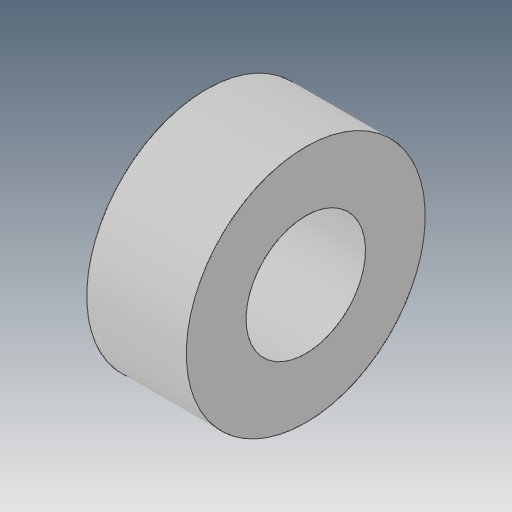
# Autodesk Inventor part: セットカラー_6mm
Saved by Autodesk Inventor 2019 (Build 230136000, 136)
## iProperties
Created: 2020-10-25
Part Number: セットカラー_6mm
Material: 一般
Document SubType Name: Modeling
Designer: zhept
Density: 1 g/cm^3
Appearance: 既定
Mass: 0.424115 g
Surface Area: 4.52389 cm^2
Volume: 0.424115 cm^3
Author: zhept
Autodesk Inventor part; units mm, degrees
ref_plane "YZ Plane" through (0, 0, 0) normal (1, 0, 0) x (0, 1, 0)
ref_plane "XZ Plane" through (0, 0, 0) normal (0, 1, 0) x (-1, 0, 0)
ref_plane "XY Plane" through (0, 0, 0) normal (0, 0, 1) x (1, 0, 0)
sketch "スケッチ1" plane through (0, 0, 0) normal (1, 0, 0) x (0, 1, 0)
  circle A0 centre (0, 0) radius 3
  circle A1 centre (0, 0) radius 6
  dimension "d0" = 6
  dimension "d1" = 12
  constraints: 2 centre point, 2 coincident
  measures "d0" diameter of A0
  measures "d1" diameter of A1
extrude "押し出し1" add sketch "スケッチ1" along normal blind 5
